Autodesk Fusion 360 part; units mm, degrees
(part 2 of 8)
  line L10 (6.9913, -88.2838) -> (6.7749, -88.3028)
  line L11 (6.7749, -88.3028) -> (7.0246, -88.3098)
  spline S251 degree 3 poles (7.0246, -88.3098) (7.1657, -88.3126) (7.2814, -88.3135) (7.2879, -88.3052) knots 0 0 0 0 1 1 1 1
  spline S252 degree 3 poles (7.2879, -88.3052) (7.2923, -88.2996) (7.2762, -88.2915) (7.2558, -88.289) knots 0 0 0 0 1 1 1 1
  spline S253 degree 3 poles (7.2558, -88.289) (7.1973, -88.2836) (7.3015, -88.1904) (7.3872, -88.1723) knots 0 0 0 0 1 1 1 1
  spline S254 degree 3 poles (7.3872, -88.1723) (7.4801, -88.1509) (7.4384, -88.1183) (7.3122, -88.1137) knots 0 0 0 0 1 1 1 1
  spline S255 degree 3 poles (7.3122, -88.1137) (7.1931, -88.1057) (7.1743, -88.0552) (7.2799, -88.0347) knots 0 0 0 0 1 1 1 1
  spline S256 degree 3 poles (7.2799, -88.0347) (7.3507, -88.0185) (7.348, -88.0163) (7.2641, -88.009) knots 0 0 0 0 1 1 1 1
  spline S257 degree 3 poles (7.2641, -88.009) (7.2029, -88.0014) (7.1744, -88.015) (7.178, -88.0447) knots 0 0 0 0 1 1 1 1
  spline S258 degree 3 poles (7.178, -88.0447) (7.1878, -88.1239) (7.1686, -88.1313) (6.9508, -88.1178) knots 0 0 0 0 1 1 1 1
  spline S259 degree 3 poles (6.9508, -88.1178) (6.6934, -88.1092) (6.6114, -88.1168) (6.6162, -88.1564) knots 0 0 0 0 1 1 1 1
  spline S260 degree 3 poles (6.6162, -88.1564) (6.618, -88.1713) (6.5929, -88.1919) (6.5589, -88.2012) knots 0 0 0 0 1 1 1 1
  spline S261 degree 3 poles (6.5589, -88.2012) (6.5121, -88.2094) (6.5084, -88.2199) (6.5306, -88.2373) knots 0 0 0 0 1 1 1 1
  spline S262 degree 3 poles (3.0505, -92.9095) (3.0667, -92.9804) (3.0716, -92.9798) (3.0703, -92.9071) knots 0 0 0 0 1 1 1 1
  spline S263 degree 3 poles (3.0703, -92.9071) (3.0703, -92.8668) (3.0655, -92.8272) (3.0599, -92.8229) knots 0 0 0 0 1 1 1 1
  spline S264 degree 3 poles (3.0599, -92.8229) (3.0377, -92.8055) (3.0342, -92.8386) (3.0505, -92.9095) knots 0 0 0 0 1 1 1 1
  spline S265 degree 3 poles (6.6279, -88.3133) (6.6335, -88.3177) (6.6731, -88.3128) (6.7143, -88.3002) knots 0 0 0 0 1 1 1 1
  spline S266 degree 3 poles (6.7143, -88.3002) (6.783, -88.2867) (6.7824, -88.2818) (6.7097, -88.2832) knots 0 0 0 0 1 1 1 1
  spline S267 degree 3 poles (6.7097, -88.2832) (6.637, -88.2846) (6.6057, -88.2959) (6.6279, -88.3133) knots 0 0 0 0 1 1 1 1
  spline S268 degree 3 poles (3.0531, -93.1354) (3.0693, -93.2062) (3.0742, -93.2056) (3.0729, -93.1329) knots 0 0 0 0 1 1 1 1
  spline S269 degree 3 poles (3.0729, -93.1329) (3.0729, -93.0927) (3.0681, -93.0531) (3.0625, -93.0487) knots 0 0 0 0 1 1 1 1
  spline S270 degree 3 poles (3.0625, -93.0487) (3.0403, -93.0314) (3.0368, -93.0645) (3.0531, -93.1354) knots 0 0 0 0 1 1 1 1
  line L12 (3.0526, -93.3365) -> (3.0753, -93.4392)
  line L13 (3.0753, -93.4392) -> (3.0724, -93.334)
  spline S271 degree 3 poles (3.0724, -93.334) (3.068, -93.2366) (3.0588, -93.2025) (3.0414, -93.2248) knots 0 0 0 0 1 1 1 1
  spline S272 degree 3 poles (3.0414, -93.2248) (3.0371, -93.2303) (3.0431, -93.2798) (3.0526, -93.3365) knots 0 0 0 0 1 1 1 1
  line L14 (3.0552, -93.5623) -> (3.0779, -93.6651)
  line L15 (3.0779, -93.6651) -> (3.075, -93.5599)
  spline S273 degree 3 poles (3.075, -93.5599) (3.0706, -93.4624) (3.0614, -93.4284) (3.044, -93.4506) knots 0 0 0 0 1 1 1 1
  spline S274 degree 3 poles (3.044, -93.4506) (3.0397, -93.4562) (3.0457, -93.5057) (3.0552, -93.5623) knots 0 0 0 0 1 1 1 1
  spline S275 degree 3 poles (7.3742, -88.0458) (7.3798, -88.0501) (7.4194, -88.0452) (7.4606, -88.0326) knots 0 0 0 0 1 1 1 1
  spline S276 degree 3 poles (7.4606, -88.0326) (7.5293, -88.0192) (7.5287, -88.0142) (7.456, -88.0156) knots 0 0 0 0 1 1 1 1
  spline S277 degree 3 poles (7.456, -88.0156) (7.3832, -88.017) (7.352, -88.0284) (7.3742, -88.0458) knots 0 0 0 0 1 1 1 1
  spline S278 degree 3 poles (8.0494, -87.4451) (8.5983, -87.4531) (9.0302, -87.4504) (9.0389, -87.4392) knots 0 0 0 0 1 1 1 1
  spline S279 degree 3 poles (9.0389, -87.4392) (9.0519, -87.4226) (8.2342, -87.4149) (8.0151, -87.4317) knots 0 0 0 0 1 1 1 1
  spline S280 degree 3 poles (8.0151, -87.4317) (7.8582, -87.4435) (7.8582, -87.4435) (8.0494, -87.4451) knots 0 0 0 0 1 1 1 1
  spline S281 degree 3 poles (3.0548, -93.7635) (3.071, -93.8343) (3.076, -93.8337) (3.0746, -93.761) knots 0 0 0 0 1 1 1 1
  spline S282 degree 3 poles (3.0746, -93.761) (3.0747, -93.7208) (3.0698, -93.6812) (3.0642, -93.6768) knots 0 0 0 0 1 1 1 1
  spline S283 degree 3 poles (3.0642, -93.6768) (3.042, -93.6595) (3.0385, -93.6926) (3.0548, -93.7635) knots 0 0 0 0 1 1 1 1
  spline S284 degree 3 poles (7.3295, -88.2347) (7.3657, -88.2629) (7.5307, -88.2351) (7.5264, -88.2005) knots 0 0 0 0 1 1 1 1
  spline S285 degree 3 poles (7.5264, -88.2005) (7.5246, -88.1856) (7.5586, -88.1764) (7.601, -88.1737) knots 0 0 0 0 1 1 1 1
  spline S286 degree 3 poles (7.601, -88.1737) (7.6737, -88.1723) (7.6743, -88.1773) (7.6056, -88.1907) knots 0 0 0 0 1 1 1 1
  spline S287 degree 3 poles (7.6056, -88.1907) (7.5645, -88.2033) (7.5387, -88.2191) (7.5499, -88.2278) knots 0 0 0 0 1 1 1 1
  spline S288 degree 3 poles (7.5499, -88.2278) (7.5888, -88.2582) (7.9208, -88.24) (7.9243, -88.2069) knots 0 0 0 0 1 1 1 1
  spline S289 degree 3 poles (7.9243, -88.2069) (7.9274, -88.1915) (7.9729, -88.1733) (8.0308, -88.1737) knots 0 0 0 0 1 1 1 1
  line L16 (8.0308, -88.1737) -> (8.1332, -88.1687)
  line L17 (8.1332, -88.1687) -> (8.0326, -88.1886)
  spline S290 degree 3 poles (8.0326, -88.1886) (7.9738, -88.2008) (7.941, -88.2199) (7.9576, -88.233) knots 0 0 0 0 1 1 1 1
  spline S291 degree 3 poles (7.9576, -88.233) (7.9938, -88.2612) (8.1588, -88.2334) (8.1545, -88.1988) knots 0 0 0 0 1 1 1 1
  spline S292 degree 3 poles (8.1545, -88.1988) (8.1527, -88.1839) (8.1867, -88.1747) (8.2291, -88.172) knots 0 0 0 0 1 1 1 1
  spline S293 degree 3 poles (8.2291, -88.172) (8.3018, -88.1706) (8.3025, -88.1756) (8.2337, -88.189) knots 0 0 0 0 1 1 1 1
  spline S294 degree 3 poles (8.2337, -88.189) (8.1415, -88.2154) (8.1844, -88.2579) (8.28, -88.2386) knots 0 0 0 0 1 1 1 1
  spline S295 degree 3 poles (8.28, -88.2386) (8.3169, -88.2316) (8.3376, -88.2165) (8.3265, -88.2078) knots 0 0 0 0 1 1 1 1
  spline S296 degree 3 poles (8.3265, -88.2078) (8.3154, -88.1991) (8.3362, -88.184) (8.373, -88.177) knots 0 0 0 0 1 1 1 1
  spline S297 degree 3 poles (8.373, -88.177) (8.5247, -88.1433) (8.354, -88.1039) (8.0885, -88.1114) knots 0 0 0 0 1 1 1 1
  spline S298 degree 3 poles (8.0885, -88.1114) (7.5476, -88.1275) (7.4678, -88.1323) (7.4708, -88.157) knots 0 0 0 0 1 1 1 1
  spline S299 degree 3 poles (7.4708, -88.157) (7.4726, -88.1719) (7.4348, -88.1916) (7.3853, -88.1977) knots 0 0 0 0 1 1 1 1
  spline S300 degree 3 poles (7.3853, -88.1977) (7.3386, -88.2059) (7.3129, -88.2217) (7.3295, -88.2347) knots 0 0 0 0 1 1 1 1
  spline S301 degree 3 poles (7.8269, -88.1711) (7.8996, -88.1697) (7.9002, -88.1747) (7.8315, -88.1881) knots 0 0 0 0 1 1 1 1
  spline S302 degree 3 poles (7.8315, -88.1881) (7.7903, -88.2007) (7.7507, -88.2056) (7.7452, -88.2013) knots 0 0 0 0 1 1 1 1
  spline S303 degree 3 poles (7.7452, -88.2013) (7.7229, -88.1839) (7.7542, -88.1725) (7.8269, -88.1711) knots 0 0 0 0 1 1 1 1
  spline S304 degree 3 poles (4.7594, -91.5988) (4.7733, -91.6097) (4.798, -91.6067) (4.8089, -91.5928) knots 0 0 0 0 1 1 1 1
  spline S305 degree 3 poles (4.8089, -91.5928) (4.8219, -91.5761) (4.8167, -91.5541) (4.8028, -91.5433) knots 0 0 0 0 1 1 1 1
  spline S306 degree 3 poles (4.8028, -91.5433) (4.7861, -91.5302) (4.7663, -91.5327) (4.7533, -91.5493) knots 0 0 0 0 1 1 1 1
  spline S307 degree 3 poles (4.7533, -91.5493) (4.7424, -91.5632) (4.7427, -91.5858) (4.7594, -91.5988) knots 0 0 0 0 1 1 1 1
  spline S308 degree 3 poles (7.5506, -88.0492) (7.5561, -88.0536) (7.5957, -88.0487) (7.6369, -88.0361) knots 0 0 0 0 1 1 1 1
  spline S309 degree 3 poles (7.6369, -88.0361) (7.7056, -88.0227) (7.705, -88.0177) (7.6323, -88.0191) knots 0 0 0 0 1 1 1 1
  spline S310 degree 3 poles (7.6323, -88.0191) (7.5596, -88.0205) (7.5283, -88.0319) (7.5506, -88.0492) knots 0 0 0 0 1 1 1 1
  spline S311 degree 3 poles (3.0513, -93.9398) (3.0675, -94.0107) (3.0725, -94.0101) (3.0711, -93.9374) knots 0 0 0 0 1 1 1 1
  spline S312 degree 3 poles (3.0711, -93.9374) (3.0712, -93.8972) (3.0663, -93.8575) (3.0608, -93.8532) knots 0 0 0 0 1 1 1 1
  spline S313 degree 3 poles (3.0608, -93.8532) (3.0385, -93.8358) (3.0351, -93.8689) (3.0513, -93.9398) knots 0 0 0 0 1 1 1 1
  spline S314 degree 3 poles (6.5586, -89.4679) (6.5725, -89.4787) (6.5973, -89.4757) (6.6103, -89.459) knots 0 0 0 0 1 1 1 1
  spline S315 degree 3 poles (6.6103, -89.459) (6.6211, -89.4451) (6.6116, -89.4287) (6.5912, -89.4262) knots 0 0 0 0 1 1 1 1
  spline S316 degree 3 poles (6.5912, -89.4262) (6.568, -89.4215) (6.546, -89.4267) (6.5395, -89.435) knots 0 0 0 0 1 1 1 1
  spline S317 degree 3 poles (6.5395, -89.435) (6.5351, -89.4406) (6.5419, -89.4548) (6.5586, -89.4679) knots 0 0 0 0 1 1 1 1
  line L18 (3.0509, -94.1409) -> (3.0735, -94.2437)
  line L19 (3.0735, -94.2437) -> (3.0707, -94.1385)
  spline S318 degree 3 poles (3.0707, -94.1385) (3.0661, -94.0812) (3.0601, -94.0317) (3.0545, -94.0274) knots 0 0 0 0 1 1 1 1
  spline S319 degree 3 poles (3.0545, -94.0274) (3.0323, -94.01) (3.0316, -94.0453) (3.0509, -94.1409) knots 0 0 0 0 1 1 1 1
  spline S320 degree 3 poles (7.7764, -88.0466) (7.782, -88.051) (7.8216, -88.0461) (7.8628, -88.0335) knots 0 0 0 0 1 1 1 1
  spline S321 degree 3 poles (7.8628, -88.0335) (7.9315, -88.02) (7.9309, -88.0151) (7.8582, -88.0165) knots 0 0 0 0 1 1 1 1
  spline S322 degree 3 poles (7.8582, -88.0165) (7.7855, -88.0179) (7.7542, -88.0293) (7.7764, -88.0466) knots 0 0 0 0 1 1 1 1
  spline S323 degree 3 poles (6.2415, -90.1602) (6.2554, -90.1711) (6.2801, -90.1681) (6.2932, -90.1514) knots 0 0 0 0 1 1 1 1
  spline S324 degree 3 poles (6.2932, -90.1514) (6.304, -90.1375) (6.2945, -90.1211) (6.2741, -90.1185) knots 0 0 0 0 1 1 1 1
  spline S325 degree 3 poles (6.2741, -90.1185) (6.2509, -90.1139) (6.2289, -90.1191) (6.2224, -90.1274) knots 0 0 0 0 1 1 1 1
  spline S326 degree 3 poles (6.2224, -90.1274) (6.218, -90.133) (6.2248, -90.1472) (6.2415, -90.1602) knots 0 0 0 0 1 1 1 1
  line L20 (3.0535, -94.3668) -> (3.0761, -94.4696)
  line L21 (3.0761, -94.4696) -> (3.0733, -94.3644)
  spline S327 degree 3 poles (3.0733, -94.3644) (3.0688, -94.2669) (3.0596, -94.2328) (3.0423, -94.2551) knots 0 0 0 0 1 1 1 1
  spline S328 degree 3 poles (3.0423, -94.2551) (3.0379, -94.2606) (3.044, -94.3102) (3.0535, -94.3668) knots 0 0 0 0 1 1 1 1
  spline S329 degree 3 poles (5.2813, -91.4694) (5.2869, -91.4738) (5.3265, -91.4689) (5.3677, -91.4563) knots 0 0 0 0 1 1 1 1
  spline S330 degree 3 poles (5.3677, -91.4563) (5.4364, -91.4428) (5.4358, -91.4379) (5.3631, -91.4393) knots 0 0 0 0 1 1 1 1
  spline S331 degree 3 poles (5.3631, -91.4393) (5.2904, -91.4407) (5.2591, -91.452) (5.2813, -91.4694) knots 0 0 0 0 1 1 1 1
  spline S332 degree 3 poles (3.053, -94.5679) (3.0693, -94.6388) (3.0742, -94.6382) (3.0728, -94.5655) knots 0 0 0 0 1 1 1 1
  spline S333 degree 3 poles (3.0728, -94.5655) (3.0729, -94.5253) (3.0681, -94.4856) (3.0625, -94.4813) knots 0 0 0 0 1 1 1 1
  spline S334 degree 3 poles (3.0625, -94.4813) (3.0403, -94.4639) (3.0368, -94.497) (3.053, -94.5679) knots 0 0 0 0 1 1 1 1
  spline S335 degree 3 poles (7.913, -88.4219) (7.9835, -88.4233) (8.0485, -88.4204) (8.0529, -88.4148) knots 0 0 0 0 1 1 1 1
  spline S336 degree 3 poles (8.0529, -88.4148) (8.0594, -88.4065) (8.0074, -88.3927) (7.9412, -88.3858) knots 0 0 0 0 1 1 1 1
  spline S337 degree 3 poles (7.9412, -88.3858) (7.8744, -88.3739) (7.8122, -88.379) (7.8014, -88.3929) knots 0 0 0 0 1 1 1 1
  spline S338 degree 3 poles (7.8014, -88.3929) (7.7905, -88.4068) (7.8397, -88.4184) (7.913, -88.4219) knots 0 0 0 0 1 1 1 1
  spline S339 degree 3 poles (8.1787, -88.0475) (8.1842, -88.0519) (8.2238, -88.047) (8.265, -88.0344) knots 0 0 0 0 1 1 1 1
  spline S340 degree 3 poles (8.265, -88.0344) (8.3337, -88.0209) (8.3331, -88.016) (8.2604, -88.0174) knots 0 0 0 0 1 1 1 1
  spline S341 degree 3 poles (8.2604, -88.0174) (8.1877, -88.0188) (8.1564, -88.0301) (8.1787, -88.0475) knots 0 0 0 0 1 1 1 1
  spline S342 degree 3 poles (3.0526, -94.769) (3.0642, -94.8229) (3.0744, -94.8443) (3.0785, -94.8161) knots 0 0 0 0 1 1 1 1
  spline S343 degree 3 poles (3.0785, -94.8161) (3.0819, -94.783) (3.117, -94.7611) (3.1671, -94.76) knots 0 0 0 0 1 1 1 1
  spline S344 degree 3 poles (3.1671, -94.76) (3.2475, -94.7602) (3.2447, -94.758) (3.1646, -94.7402) knots 0 0 0 0 1 1 1 1
  spline S345 degree 3 poles (3.1646, -94.7402) (3.1183, -94.7308) (3.0722, -94.7038) (3.0648, -94.6846) knots 0 0 0 0 1 1 1 1
  spline S346 degree 3 poles (3.0648, -94.6846) (3.0387, -94.6149) (3.0321, -94.6635) (3.0526, -94.769) knots 0 0 0 0 1 1 1 1
  spline S347 degree 3 poles (7.786, -88.6361) (7.7999, -88.6469) (7.833, -88.6504) (7.8522, -88.643) knots 0 0 0 0 1 1 1 1
  spline S348 degree 3 poles (7.8522, -88.643) (7.8735, -88.6329) (7.8794, -88.6196) (7.8628, -88.6065) knots 0 0 0 0 1 1 1 1
  spline S349 degree 3 poles (7.8628, -88.6065) (7.8489, -88.5957) (7.8179, -88.5894) (7.7966, -88.5996) knots 0 0 0 0 1 1 1 1
  spline S350 degree 3 poles (7.7966, -88.5996) (7.7774, -88.607) (7.7693, -88.623) (7.786, -88.6361) knots 0 0 0 0 1 1 1 1
  spline S351 degree 3 poles (3.0521, -94.9701) (3.0684, -95.041) (3.0733, -95.0404) (3.0719, -94.9677) knots 0 0 0 0 1 1 1 1
  spline S352 degree 3 poles (3.0719, -94.9677) (3.072, -94.9275) (3.0672, -94.8879) (3.0616, -94.8835) knots 0 0 0 0 1 1 1 1
  spline S353 degree 3 poles (3.0616, -94.8835) (3.0394, -94.8662) (3.0359, -94.8993) (3.0521, -94.9701) knots 0 0 0 0 1 1 1 1
  spline S354 degree 3 poles (8.4045, -88.0449) (8.4101, -88.0492) (8.4497, -88.0444) (8.4909, -88.0318) knots 0 0 0 0 1 1 1 1
  spline S355 degree 3 poles (8.4909, -88.0318) (8.5596, -88.0183) (8.559, -88.0134) (8.4863, -88.0148) knots 0 0 0 0 1 1 1 1
  spline S356 degree 3 poles (8.4863, -88.0148) (8.4136, -88.0162) (8.3823, -88.0275) (8.4045, -88.0449) knots 0 0 0 0 1 1 1 1
  spline S357 degree 3 poles (8.3515, -88.2273) (8.3877, -88.2556) (8.9505, -88.2342) (8.9546, -88.2061) knots 0 0 0 0 1 1 1 1
  spline S358 degree 3 poles (8.9546, -88.2061) (8.955, -88.1884) (8.9934, -88.1737) (9.0364, -88.1759) knots 0 0 0 0 1 1 1 1
  spline S359 degree 3 poles (9.0364, -88.1759) (9.1063, -88.1724) (9.1069, -88.1773) (9.0382, -88.1908) knots 0 0 0 0 1 1 1 1
  spline S360 degree 3 poles (9.0382, -88.1908) (8.9921, -88.204) (8.9741, -88.2213) (8.9908, -88.2343) knots 0 0 0 0 1 1 1 1
  spline S361 degree 3 poles (8.9908, -88.2343) (9.0213, -88.2582) (9.1071, -88.2401) (9.1397, -88.1984) knots 0 0 0 0 1 1 1 1
  spline S362 degree 3 poles (9.1397, -88.1984) (9.1483, -88.1873) (9.2474, -88.1751) (9.3603, -88.1738) knots 0 0 0 0 1 1 1 1
  line L22 (9.3603, -88.1738) -> (9.5614, -88.1743)
  line L23 (9.5614, -88.1743) -> (9.3473, -88.1905)
  spline S363 degree 3 poles (9.3473, -88.1905) (9.0808, -88.2107) (9.1055, -88.2479) (9.376, -88.2398) knots 0 0 0 0 1 1 1 1
  spline S364 degree 3 poles (9.376, -88.2398) (9.4988, -88.2373) (9.5838, -88.2545) (9.5952, -88.2857) knots 0 0 0 0 1 1 1 1
  spline S365 degree 3 poles (9.5952, -88.2857) (9.606, -88.3121) (9.6165, -88.3158) (9.6113, -88.2938) knots 0 0 0 0 1 1 1 1
  spline S366 degree 3 poles (9.6113, -88.2938) (9.611, -88.2712) (9.6482, -88.2466) (9.6977, -88.2405) knots 0 0 0 0 1 1 1 1
  spline S367 degree 3 poles (9.6977, -88.2405) (9.7445, -88.2322) (9.7702, -88.2165) (9.7591, -88.2078) knots 0 0 0 0 1 1 1 1
  spline S368 degree 3 poles (9.7591, -88.2078) (9.748, -88.1991) (9.7786, -88.1828) (9.8303, -88.1739) knots 0 0 0 0 1 1 1 1
  spline S369 degree 3 poles (9.8303, -88.1739) (9.9755, -88.1486) (9.888, -88.1116) (9.7085, -88.1236) knots 0 0 0 0 1 1 1 1
  spline S370 degree 3 poles (9.7085, -88.1236) (9.6209, -88.1268) (9.5405, -88.1266) (9.5294, -88.1179) knots 0 0 0 0 1 1 1 1
  spline S371 degree 3 poles (9.5294, -88.1179) (9.5183, -88.1092) (9.4802, -88.1063) (9.4455, -88.1106) knots 0 0 0 0 1 1 1 1
  spline S372 degree 3 poles (9.4455, -88.1106) (9.4109, -88.1149) (9.3057, -88.1177) (9.2098, -88.1144) knots 0 0 0 0 1 1 1 1
  spline S373 degree 3 poles (9.2098, -88.1144) (9.1166, -88.1133) (8.974, -88.1182) (8.8969, -88.1252) knots 0 0 0 0 1 1 1 1
  spline S374 degree 3 poles (8.8969, -88.1252) (8.8171, -88.13) (8.7416, -88.1292) (8.7277, -88.1183) knots 0 0 0 0 1 1 1 1
  spline S375 degree 3 poles (8.7277, -88.1183) (8.7138, -88.1075) (8.694, -88.1099) (8.681, -88.1266) knots 0 0 0 0 1 1 1 1
  spline S376 degree 3 poles (8.681, -88.1266) (8.6701, -88.1405) (8.688, -88.1634) (8.7217, -88.1718) knots 0 0 0 0 1 1 1 1
  spline S377 degree 3 poles (8.7217, -88.1718) (8.756, -88.1852) (8.7749, -88.1955) (8.7622, -88.1945) knots 0 0 0 0 1 1 1 1
  spline S378 degree 3 poles (8.7622, -88.1945) (8.5722, -88.2028) (8.5187, -88.1968) (8.5917, -88.1777) knots 0 0 0 0 1 1 1 1
  spline S379 degree 3 poles (8.5917, -88.1777) (8.6456, -88.1661) (8.6565, -88.1522) (8.6342, -88.1348) knots 0 0 0 0 1 1 1 1
  spline S380 degree 3 poles (8.6342, -88.1348) (8.5897, -88.1001) (8.4461, -88.1177) (8.451, -88.1573) knots 0 0 0 0 1 1 1 1
  spline S381 degree 3 poles (8.451, -88.1573) (8.4528, -88.1722) (8.4277, -88.1929) (8.3937, -88.2021) knots 0 0 0 0 1 1 1 1
  spline S382 degree 3 poles (8.3937, -88.2021) (8.3618, -88.2085) (8.3432, -88.2208) (8.3515, -88.2273) knots 0 0 0 0 1 1 1 1
  spline S383 degree 3 poles (9.7263, -88.1867) (9.7281, -88.2016) (9.6885, -88.2064) (9.64, -88.1998) knots 0 0 0 0 1 1 1 1
  spline S384 degree 3 poles (9.64, -88.1998) (9.5534, -88.1904) (9.5555, -88.1876) (9.6369, -88.1751) knots 0 0 0 0 1 1 1 1
  spline S385 degree 3 poles (9.6369, -88.1751) (9.6864, -88.169) (9.7273, -88.174) (9.7263, -88.1867) knots 0 0 0 0 1 1 1 1
  line L24 (3.0517, -95.1713) -> (3.0744, -95.274)
  line L25 (3.0744, -95.274) -> (3.0715, -95.1688)
  spline S386 degree 3 poles (3.0715, -95.1688) (3.0671, -95.0713) (3.0579, -95.0373) (3.0405, -95.0595) knots 0 0 0 0 1 1 1 1
  spline S387 degree 3 poles (3.0405, -95.0595) (3.0362, -95.0651) (3.0422, -95.1146) (3.0517, -95.1713) knots 0 0 0 0 1 1 1 1
  spline S388 degree 3 poles (8.6304, -88.0423) (8.636, -88.0466) (8.6756, -88.0418) (8.7168, -88.0292) knots 0 0 0 0 1 1 1 1
  spline S389 degree 3 poles (8.7168, -88.0292) (8.7855, -88.0157) (8.7849, -88.0108) (8.7122, -88.0122) knots 0 0 0 0 1 1 1 1
  spline S390 degree 3 poles (8.7122, -88.0122) (8.6394, -88.0135) (8.6082, -88.0249) (8.6304, -88.0423) knots 0 0 0 0 1 1 1 1
  spline S391 degree 3 poles (9.1636, -87.4516) (9.2159, -87.4477) (9.2626, -87.4394) (9.2691, -87.4311) knots 0 0 0 0 1 1 1 1
  spline S392 degree 3 poles (9.2691, -87.4311) (9.2756, -87.4227) (9.2376, -87.4199) (9.1853, -87.4238) knots 0 0 0 0 1 1 1 1
  spline S393 degree 3 poles (9.1853, -87.4238) (9.133, -87.4277) (9.0862, -87.4359) (9.0797, -87.4443) knots 0 0 0 0 1 1 1 1
  spline S394 degree 3 poles (9.0797, -87.4443) (9.0732, -87.4526) (9.1113, -87.4555) (9.1636, -87.4516) knots 0 0 0 0 1 1 1 1
  spline S395 degree 3 poles (3.0513, -95.3724) (3.0675, -95.4433) (3.0725, -95.4426) (3.0711, -95.3699) knots 0 0 0 0 1 1 1 1
  spline S396 degree 3 poles (3.0711, -95.3699) (3.0712, -95.3297) (3.0663, -95.2901) (3.0607, -95.2858) knots 0 0 0 0 1 1 1 1
  spline S397 degree 3 poles (3.0607, -95.2858) (3.0385, -95.2684) (3.035, -95.3015) (3.0513, -95.3724) knots 0 0 0 0 1 1 1 1
  line L26 (3.0508, -95.5735) -> (3.0735, -95.6763)
  line L27 (3.0735, -95.6763) -> (3.0706, -95.571)
  spline S398 degree 3 poles (3.0706, -95.571) (3.0662, -95.4736) (3.057, -95.4395) (3.0396, -95.4618) knots 0 0 0 0 1 1 1 1
  spline S399 degree 3 poles (3.0396, -95.4618) (3.0353, -95.4673) (3.0414, -95.5168) (3.0508, -95.5735) knots 0 0 0 0 1 1 1 1
  spline S400 degree 3 poles (9.563, -87.4503) (9.7162, -87.4491) (9.861, -87.4413) (9.883, -87.4361) knots 0 0 0 0 1 1 1 1
  spline S401 degree 3 poles (9.883, -87.4361) (9.9043, -87.426) (9.7957, -87.4217) (9.6398, -87.4207) knots 0 0 0 0 1 1 1 1
  spline S402 degree 3 poles (9.6398, -87.4207) (9.4866, -87.422) (9.3418, -87.4297) (9.3199, -87.4349) knots 0 0 0 0 1 1 1 1
  spline S403 degree 3 poles (9.3199, -87.4349) (9.2985, -87.4451) (9.4071, -87.4493) (9.563, -87.4503) knots 0 0 0 0 1 1 1 1
  spline S404 degree 3 poles (6.5564, -91.1897) (6.6087, -91.1858) (6.6554, -91.1776) (6.6619, -91.1692) knots 0 0 0 0 1 1 1 1
  spline S405 degree 3 poles (6.6619, -91.1692) (6.6685, -91.1609) (6.6304, -91.158) (6.5781, -91.1619) knots 0 0 0 0 1 1 1 1
  spline S406 degree 3 poles (6.5781, -91.1619) (6.5258, -91.1658) (6.4791, -91.1741) (6.4726, -91.1824) knots 0 0 0 0 1 1 1 1
  spline S407 degree 3 poles (6.4726, -91.1824) (6.466, -91.1908) (6.5041, -91.1936) (6.5564, -91.1897) knots 0 0 0 0 1 1 1 1
  line L28 (3.0511, -95.8826) -> (3.0643, -96.072)
  line L29 (3.0643, -96.072) -> (3.0687, -95.8829)
  spline S408 degree 3 poles (3.0687, -95.8829) (3.0718, -95.7242) (3.0639, -95.6598) (3.0444, -95.6849) knots 0 0 0 0 1 1 1 1
  spline S409 degree 3 poles (3.0444, -95.6849) (3.0401, -95.6904) (3.0433, -95.778) (3.0511, -95.8826) knots 0 0 0 0 1 1 1 1
  spline S410 degree 3 poles (7.6583, -89.9913) (7.5611, -90.1616) (7.4813, -90.3096) (7.4853, -90.3217) knots 0 0 0 0 1 1 1 1
  spline S411 degree 3 poles (7.4853, -90.3217) (7.4898, -90.3789) (7.5413, -90.3073) (7.7112, -89.9924) knots 0 0 0 0 1 1 1 1
  spline S412 degree 3 poles (7.7112, -89.9924) (7.8137, -89.8038) (7.9144, -89.6407) (7.9363, -89.6355) knots 0 0 0 0 1 1 1 1
  spline S413 degree 3 poles (7.9363, -89.6355) (7.9577, -89.6253) (7.9543, -89.6182) (7.9289, -89.6163) knots 0 0 0 0 1 1 1 1
  spline S414 degree 3 poles (7.9289, -89.6163) (7.9008, -89.6122) (7.8701, -89.6285) (7.8571, -89.6452) knots 0 0 0 0 1 1 1 1
  spline S415 degree 3 poles (7.8571, -89.6452) (7.8447, -89.6668) (7.7555, -89.821) (7.6583, -89.9913) knots 0 0 0 0 1 1 1 1
  spline S416 degree 3 poles (8.9103, -88.5206) (8.9808, -88.522) (9.0437, -88.5219) (9.048, -88.5163) knots 0 0 0 0 1 1 1 1
  spline S417 degree 3 poles (9.048, -88.5163) (9.0523, -88.5107) (9.0026, -88.4942) (8.9385, -88.4845) knots 0 0 0 0 1 1 1 1
  spline S418 degree 3 poles (8.9385, -88.4845) (8.8717, -88.4726) (8.8117, -88.4749) (8.7987, -88.4916) knots 0 0 0 0 1 1 1 1
  spline S419 degree 3 poles (8.7987, -88.4916) (8.7878, -88.5055) (8.8348, -88.5199) (8.9103, -88.5206) knots 0 0 0 0 1 1 1 1
  spline S420 degree 3 poles (8.2573, -89.2819) (8.2809, -89.269) (8.2976, -89.2418) (8.2958, -89.2269) knots 0 0 0 0 1 1 1 1
  spline S421 degree 3 poles (8.2958, -89.2269) (8.2962, -89.2093) (8.2748, -89.2194) (8.2537, -89.2522) knots 0 0 0 0 1 1 1 1
  spline S422 degree 3 poles (8.2537, -89.2522) (8.2298, -89.2828) (8.2316, -89.2976) (8.2573, -89.2819) knots 0 0 0 0 1 1 1 1
  line L30 (3.0525, -96.2016) -> (3.0752, -96.3044)
  line L31 (3.0752, -96.3044) -> (3.0724, -96.1992)
  spline S423 degree 3 poles (3.0724, -96.1992) (3.0679, -96.1017) (3.0587, -96.0676) (3.0413, -96.0899) knots 0 0 0 0 1 1 1 1
  spline S424 degree 3 poles (3.0413, -96.0899) (3.037, -96.0954) (3.0431, -96.1449) (3.0525, -96.2016) knots 0 0 0 0 1 1 1 1
  spline S425 degree 3 poles (7.0702, -91.0764) (7.1374, -91.0706) (7.1962, -91.0584) (7.2006, -91.0528) knots 0 0 0 0 1 1 1 1
  spline S426 degree 3 poles (7.2006, -91.0528) (7.2071, -91.0445) (7.1591, -91.0428) (7.092, -91.0486) knots 0 0 0 0 1 1 1 1
  spline S427 degree 3 poles (7.092, -91.0486) (7.0248, -91.0543) (6.966, -91.0665) (6.9617, -91.0721) knots 0 0 0 0 1 1 1 1
  spline S428 degree 3 poles (6.9617, -91.0721) (6.9551, -91.0804) (7.0031, -91.0821) (7.0702, -91.0764) knots 0 0 0 0 1 1 1 1
  spline S429 degree 3 poles (4.765, -93.9983) (4.7724, -94.0175) (4.7906, -94.0228) (4.8015, -94.0089) knots 0 0 0 0 1 1 1 1
  spline S430 degree 3 poles (4.8015, -94.0089) (4.8145, -93.9922) (4.8115, -93.9675) (4.7976, -93.9566) knots 0 0 0 0 1 1 1 1
  spline S431 degree 3 poles (4.7976, -93.9566) (4.7809, -93.9436) (4.7654, -93.9405) (4.7611, -93.946) knots 0 0 0 0 1 1 1 1
  spline S432 degree 3 poles (4.7611, -93.946) (4.7546, -93.9544) (4.7548, -93.9769) (4.765, -93.9983) knots 0 0 0 0 1 1 1 1
  spline S433 degree 3 poles (9.9779, -87.4521) (10.4408, -87.4556) (10.9145, -87.4452) (10.921, -87.4368) knots 0 0 0 0 1 1 1 1
  spline S434 degree 3 poles (10.921, -87.4368) (10.9275, -87.4285) (10.7082, -87.4228) (10.4393, -87.4231) knots 0 0 0 0 1 1 1 1
  spline S435 degree 3 poles (10.4393, -87.4231) (10.1677, -87.4213) (9.9424, -87.4288) (9.9359, -87.4372) knots 0 0 0 0 1 1 1 1
  spline S436 degree 3 poles (9.9359, -87.4372) (9.9294, -87.4455) (9.9504, -87.453) (9.9779, -87.4521) knots 0 0 0 0 1 1 1 1
  spline S437 degree 3 poles (3.0521, -96.4027) (3.0684, -96.4736) (3.0733, -96.473) (3.0719, -96.4003) knots 0 0 0 0 1 1 1 1
  spline S438 degree 3 poles (3.0719, -96.4003) (3.072, -96.36) (3.0671, -96.3204) (3.0616, -96.3161) knots 0 0 0 0 1 1 1 1
  spline S439 degree 3 poles (3.0616, -96.3161) (3.0393, -96.2987) (3.0359, -96.3318) (3.0521, -96.4027) knots 0 0 0 0 1 1 1 1
  spline S440 degree 3 poles (8.9747, -88.7992) (9.0137, -88.7894) (9.0579, -88.8016) (9.0758, -88.8245) knots 0 0 0 0 1 1 1 1
  spline S441 degree 3 poles (9.0758, -88.8245) (9.1032, -88.8639) (9.1054, -88.8611) (9.0894, -88.8128) knots 0 0 0 0 1 1 1 1
  spline S442 degree 3 poles (9.0894, -88.8128) (9.0734, -88.7645) (9.1063, -88.7454) (9.2595, -88.704) knots 0 0 0 0 1 1 1 1
  spline S443 degree 3 poles (9.2595, -88.704) (9.5474, -88.6334) (9.5546, -88.63) (9.5379, -88.617) knots 0 0 0 0 1 1 1 1
  spline S444 degree 3 poles (9.5379, -88.617) (9.5156, -88.5996) (8.945, -88.7627) (8.9233, -88.7905) knots 0 0 0 0 1 1 1 1
  spline S445 degree 3 poles (8.9233, -88.7905) (8.9125, -88.8044) (8.9357, -88.8091) (8.9747, -88.7992) knots 0 0 0 0 1 1 1 1
  spline S446 degree 3 poles (7.3691, -90.9517) (7.4127, -90.9589) (7.4529, -90.959) (7.4594, -90.9507) knots 0 0 0 0 1 1 1 1
  spline S447 degree 3 poles (7.4594, -90.9507) (7.4638, -90.9451) (7.4344, -90.9311) (7.3908, -90.9239) knots 0 0 0 0 1 1 1 1
  spline S448 degree 3 poles (7.3908, -90.9239) (7.3472, -90.9167) (7.307, -90.9166) (7.3005, -90.9249) knots 0 0 0 0 1 1 1 1
  spline S449 degree 3 poles (7.3005, -90.9249) (7.2961, -90.9305) (7.3255, -90.9445) (7.3691, -90.9517) knots 0 0 0 0 1 1 1 1
  spline S450 degree 3 poles (7.3012, -91.0329) (7.3151, -91.0438) (7.3482, -91.0473) (7.3674, -91.0399) knots 0 0 0 0 1 1 1 1
  spline S451 degree 3 poles (7.3674, -91.0399) (7.3887, -91.0297) (7.3946, -91.0164) (7.378, -91.0034) knots 0 0 0 0 1 1 1 1
  spline S452 degree 3 poles (7.378, -91.0034) (7.3641, -90.9925) (7.3331, -90.9863) (7.3118, -90.9964) knots 0 0 0 0 1 1 1 1
  spline S453 degree 3 poles (7.3118, -90.9964) (7.2926, -91.0038) (7.2845, -91.0199) (7.3012, -91.0329) knots 0 0 0 0 1 1 1 1
  spline S454 degree 3 poles (10.0458, -87.5544) (10.0767, -87.5606) (10.1114, -87.5564) (10.1222, -87.5425) knots 0 0 0 0 1 1 1 1
  spline S455 degree 3 poles (10.1222, -87.5425) (10.1353, -87.5258) (10.1164, -87.5155) (10.0762, -87.5154) knots 0 0 0 0 1 1 1 1
  spline S456 degree 3 poles (10.0762, -87.5154) (10.0387, -87.5175) (10.0041, -87.5218) (9.9997, -87.5273) knots 0 0 0 0 1 1 1 1
  spline S457 degree 3 poles (9.9997, -87.5273) (9.9954, -87.5329) (10.017, -87.5453) (10.0458, -87.5544) knots 0 0 0 0 1 1 1 1
  line L32 (3.0517, -96.6038) -> (3.0743, -96.7066)
  line L33 (3.0743, -96.7066) -> (3.0715, -96.6014)
  spline S458 degree 3 poles (3.0715, -96.6014) (3.067, -96.5441) (3.0609, -96.4946) (3.0553, -96.4903) knots 0 0 0 0 1 1 1 1
  spline S459 degree 3 poles (3.0553, -96.4903) (3.0331, -96.4729) (3.0324, -96.5082) (3.0517, -96.6038) knots 0 0 0 0 1 1 1 1
  spline S460 degree 3 poles (3.0512, -96.8049) (3.0675, -96.8758) (3.0724, -96.8752) (3.071, -96.8025) knots 0 0 0 0 1 1 1 1
  spline S461 degree 3 poles (3.071, -96.8025) (3.0711, -96.7623) (3.0663, -96.7227) (3.0607, -96.7183) knots 0 0 0 0 1 1 1 1
  spline S462 degree 3 poles (3.0607, -96.7183) (3.0385, -96.7009) (3.035, -96.734) (3.0512, -96.8049) knots 0 0 0 0 1 1 1 1
  spline S463 degree 3 poles (9.8371, -88.0449) (9.8426, -88.0493) (9.8823, -88.0444) (9.9234, -88.0318) knots 0 0 0 0 1 1 1 1
  spline S464 degree 3 poles (9.9234, -88.0318) (9.9922, -88.0184) (9.9915, -88.0134) (9.9188, -88.0148) knots 0 0 0 0 1 1 1 1
  spline S465 degree 3 poles (9.9188, -88.0148) (9.8461, -88.0162) (9.8148, -88.0276) (9.8371, -88.0449) knots 0 0 0 0 1 1 1 1
  spline S466 degree 3 poles (8.3907, -89.9994) (8.4185, -90.0211) (8.432, -90.0496) (8.4255, -90.058) knots 0 0 0 0 1 1 1 1
  spline S467 degree 3 poles (8.4255, -90.058) (8.419, -90.0663) (8.359, -90.1717) (8.291, -90.2931) knots 0 0 0 0 1 1 1 1
  spline S468 degree 3 poles (8.291, -90.2931) (8.1323, -90.5765) (8.0293, -90.9661) (8.0302, -91.2802) knots 0 0 0 0 1 1 1 1
  line L34 (8.0302, -91.2802) -> (8.0337, -91.5336)
  line L35 (8.0337, -91.5336) -> (7.9077, -91.5516)
  spline S469 degree 3 poles (7.9077, -91.5516) (7.8384, -91.5601) (7.7731, -91.5807) (7.7644, -91.5918) knots 0 0 0 0 1 1 1 1
  spline S470 degree 3 poles (7.7644, -91.5918) (7.7535, -91.6057) (7.8114, -91.6061) (7.89, -91.5914) knots 0 0 0 0 1 1 1 1
  line L36 (7.89, -91.5914) -> (8.033, -91.5689)
  line L37 (8.033, -91.5689) -> (8.1002, -91.8094)
  spline S471 degree 3 poles (8.1002, -91.8094) (8.1524, -91.989) (8.1554, -92.054) (8.1089, -92.0848) knots 0 0 0 0 1 1 1 1
  spline S472 degree 3 poles (8.1089, -92.0848) (8.0745, -92.1117) (8.0714, -92.1271) (8.0995, -92.1312) knots 0 0 0 0 1 1 1 1
  spline S473 degree 3 poles (8.0995, -92.1312) (8.1861, -92.1407) (8.2018, -92.0634) (8.1474, -91.8866) knots 0 0 0 0 1 1 1 1
  spline S474 degree 3 poles (8.1474, -91.8866) (8.0814, -91.6559) (8.0629, -91.4848) (8.0888, -91.3484) knots 0 0 0 0 1 1 1 1
  spline S475 degree 3 poles (8.0888, -91.3484) (8.0992, -91.2893) (8.0988, -91.2039) (8.0855, -91.1578) knots 0 0 0 0 1 1 1 1
  spline S476 degree 3 poles (8.0855, -91.1578) (8.0625, -91.0726) (8.1516, -90.6722) (8.1961, -90.6667) knots 0 0 0 0 1 1 1 1
  spline S477 degree 3 poles (8.1961, -90.6667) (8.211, -90.6649) (8.2194, -90.6311) (8.2167, -90.5888) knots 0 0 0 0 1 1 1 1
  spline S478 degree 3 poles (8.2167, -90.5888) (8.2168, -90.5485) (8.2672, -90.4267) (8.3371, -90.3201) knots 0 0 0 0 1 1 1 1
  line L38 (8.3371, -90.3201) -> (8.456, -90.1221)
  line L39 (8.456, -90.1221) -> (8.4579, -90.24)
  spline S479 degree 3 poles (8.4579, -90.24) (8.4577, -90.3204) (8.4192, -90.4156) (8.3341, -90.5417) knots 0 0 0 0 1 1 1 1
  spline S480 degree 3 poles (8.3341, -90.5417) (8.2658, -90.6405) (8.2136, -90.7475) (8.2179, -90.7821) knots 0 0 0 0 1 1 1 1
  spline S481 degree 3 poles (8.2179, -90.7821) (8.2255, -90.8239) (8.2342, -90.8128) (8.2675, -90.7358) knots 0 0 0 0 1 1 1 1
  spline S482 degree 3 poles (8.2675, -90.7358) (8.2933, -90.6799) (8.4233, -90.4905) (8.5629, -90.3175) knots 0 0 0 0 1 1 1 1
  spline S483 degree 3 poles (8.5629, -90.3175) (8.8003, -90.0195) (8.8319, -89.9905) (9.0887, -89.8509) knots 0 0 0 0 1 1 1 1
  spline S484 degree 3 poles (9.0887, -89.8509) (9.6001, -89.5744) (10.0678, -89.5145) (10.621, -89.6602) knots 0 0 0 0 1 1 1 1
  spline S485 degree 3 poles (10.621, -89.6602) (10.8752, -89.7245) (10.9633, -89.7665) (11.2321, -89.9496) knots 0 0 0 0 1 1 1 1
  spline S486 degree 3 poles (11.2321, -89.9496) (11.4931, -90.1312) (11.5225, -90.1452) (11.4194, -90.0422) knots 0 0 0 0 1 1 1 1
  spline S487 degree 3 poles (11.4194, -90.0422) (11.2499, -89.8695) (10.8651, -89.6629) (10.5982, -89.5977) knots 0 0 0 0 1 1 1 1
  line L40 (10.5982, -89.5977) -> (10.3756, -89.5446)
  line L41 (10.3756, -89.5446) -> (10.3755, -89.4415)
  spline S488 degree 3 poles (10.3755, -89.4415) (10.3759, -89.3837) (10.3819, -89.3302) (10.3884, -89.3218) knots 0 0 0 0 1 1 1 1
  spline S489 degree 3 poles (10.3884, -89.3218) (10.3971, -89.3107) (10.5054, -89.3326) (10.6325, -89.3647) knots 0 0 0 0 1 1 1 1
  line L42 (10.6325, -89.3647) -> (10.8635, -89.4243)
  line L43 (10.8635, -89.4243) -> (10.8663, -89.5296)
  line L44 (10.8663, -89.5296) -> (10.8664, -89.6326)
  line L45 (10.8664, -89.6326) -> (10.8858, -89.5448)
  spline S490 degree 3 poles (10.8858, -89.5448) (10.8974, -89.4956) (10.9194, -89.4502) (10.9371, -89.4505) knots 0 0 0 0 1 1 1 1
  spline S491 degree 3 poles (10.9371, -89.4505) (10.9569, -89.4481) (11.1302, -89.57) (11.3248, -89.7221) knots 0 0 0 0 1 1 1 1
  spline S492 degree 3 poles (11.3248, -89.7221) (11.5833, -89.9241) (11.6858, -90.0221) (11.6975, -90.0759) knots 0 0 0 0 1 1 1 1
  spline S493 degree 3 poles (11.6975, -90.0759) (11.7073, -90.1149) (11.718, -90.1413) (11.7246, -90.1329) knots 0 0 0 0 1 1 1 1
  spline S494 degree 3 poles (11.7246, -90.1329) (11.7311, -90.1246) (11.7894, -90.2104) (11.8535, -90.3232) knots 0 0 0 0 1 1 1 1
  spline S495 degree 3 poles (11.8535, -90.3232) (12.0064, -90.5859) (12.127, -91.0159) (12.0957, -91.1705) knots 0 0 0 0 1 1 1 1
  spline S496 degree 3 poles (12.0957, -91.1705) (12.0838, -91.2374) (12.0816, -91.2804) (12.0924, -91.2665) knots 0 0 0 0 1 1 1 1
  spline S497 degree 3 poles (12.0924, -91.2665) (12.1229, -91.2275) (12.1129, -91.5153) (12.0789, -91.6677) knots 0 0 0 0 1 1 1 1
  spline S498 degree 3 poles (12.0789, -91.6677) (12.0442, -91.8152) (12.0791, -91.8336) (12.1166, -91.6882) knots 0 0 0 0 1 1 1 1
  spline S499 degree 3 poles (12.1166, -91.6882) (12.136, -91.6004) (12.1496, -91.5887) (12.2273, -91.5867) knots 0 0 0 0 1 1 1 1
  spline S500 degree 3 poles (12.2273, -91.5867) (12.3099, -91.5841) (12.3099, -91.5841) (12.2326, -91.5684) knots 0 0 0 0 1 1 1 1
  spline S501 degree 3 poles (12.2326, -91.5684) (12.1602, -91.5522) (12.1488, -91.5209) (12.15, -91.2845) knots 0 0 0 0 1 1 1 1
  spline S502 degree 3 poles (12.15, -91.2845) (12.1485, -90.9655) (12.0435, -90.5612) (11.8894, -90.2886) knots 0 0 0 0 1 1 1 1
  spline S503 degree 3 poles (11.8894, -90.2886) (11.7375, -90.0132) (11.422, -89.6951) (11.1374, -89.5264) knots 0 0 0 0 1 1 1 1
  spline S504 degree 3 poles (11.1374, -89.5264) (10.9504, -89.4162) (10.9081, -89.3787) (10.912, -89.3279) knots 0 0 0 0 1 1 1 1
  spline S505 degree 3 poles (10.912, -89.3279) (10.9136, -89.28) (10.9108, -89.2778) (10.8915, -89.3254) knots 0 0 0 0 1 1 1 1
  spline S506 degree 3 poles (10.8915, -89.3254) (10.8638, -89.4067) (10.3879, -89.2767) (10.3946, -89.1879) knots 0 0 0 0 1 1 1 1
  spline S507 degree 3 poles (10.3946, -89.1879) (10.4018, -89.1443) (10.3885, -89.1383) (10.3452, -89.1537) knots 0 0 0 0 1 1 1 1
  spline S508 degree 3 poles (10.3452, -89.1537) (10.3139, -89.1651) (10.2845, -89.1913) (10.277, -89.2124) knots 0 0 0 0 1 1 1 1
  spline S509 degree 3 poles (10.277, -89.2124) (10.2695, -89.2334) (10.1931, -89.2453) (10.1071, -89.2408) knots 0 0 0 0 1 1 1 1
  spline S510 degree 3 poles (10.1071, -89.2408) (10.0211, -89.2362) (9.9273, -89.2302) (9.8948, -89.2316) knots 0 0 0 0 1 1 1 1
  spline S511 degree 3 poles (9.8948, -89.2316) (9.8568, -89.2288) (9.8327, -89.1965) (9.8165, -89.1257) knots 0 0 0 0 1 1 1 1
  line L46 (9.8165, -89.1257) -> (9.796, -89.0201)
  line L47 (9.796, -89.0201) -> (9.7976, -89.1154)
  spline S512 degree 3 poles (9.7976, -89.1154) (9.8015, -89.1677) (9.7955, -89.2212) (9.7868, -89.2323) knots 0 0 0 0 1 1 1 1
  spline S513 degree 3 poles (9.7868, -89.2323) (9.7673, -89.2574) (9.3097, -89.3789) (9.2931, -89.3658) knots 0 0 0 0 1 1 1 1
  spline S514 degree 3 poles (9.2931, -89.3658) (9.2847, -89.3593) (9.3027, -89.342) (9.3306, -89.3235) knots 0 0 0 0 1 1 1 1
  spline S515 degree 3 poles (9.3306, -89.3235) (9.3777, -89.2977) (9.3743, -89.2905) (9.3142, -89.2929) knots 0 0 0 0 1 1 1 1
  spline S516 degree 3 poles (9.3142, -89.2929) (9.2592, -89.2946) (9.2455, -89.3063) (9.2575, -89.3426) knots 0 0 0 0 1 1 1 1
  spline S517 degree 3 poles (9.2575, -89.3426) (9.2717, -89.376) (9.2193, -89.4201) (9.0666, -89.5068) knots 0 0 0 0 1 1 1 1
  spline S518 degree 3 poles (9.0666, -89.5068) (8.9073, -89.6017) (8.8491, -89.6189) (8.8118, -89.5808) knots 0 0 0 0 1 1 1 1
  spline S519 degree 3 poles (8.8118, -89.5808) (8.7716, -89.5405) (8.7695, -89.5432) (8.7817, -89.602) knots 0 0 0 0 1 1 1 1
  spline S520 degree 3 poles (8.7817, -89.602) (8.7887, -89.6389) (8.7685, -89.6992) (8.7325, -89.7337) knots 0 0 0 0 1 1 1 1
  spline S521 degree 3 poles (8.7325, -89.7337) (8.5027, -89.9706) (8.4569, -90.0064) (8.4037, -89.9827) knots 0 0 0 0 1 1 1 1
  spline S522 degree 3 poles (8.4037, -89.9827) (8.3505, -89.9591) (8.3484, -89.9619) (8.3907, -89.9994) knots 0 0 0 0 1 1 1 1
  spline S523 degree 3 poles (8.7689, -89.7846) (8.813, -89.7339) (8.813, -89.7339) (8.8251, -89.833) knots 0 0 0 0 1 1 1 1
  spline S524 degree 3 poles (8.8251, -89.833) (8.8389, -89.9243) (8.8199, -89.9542) (8.6729, -90.108) knots 0 0 0 0 1 1 1 1
  line L48 (8.6729, -90.108) -> (8.5079, -90.2791)
  line L49 (8.5079, -90.2791) -> (8.4924, -90.1729)
  spline S525 degree 3 poles (8.4924, -90.1729) (8.4787, -90.0816) (8.4905, -90.055) (8.6012, -89.9535) knots 0 0 0 0 1 1 1 1
  spline S526 degree 3 poles (8.6012, -89.9535) (8.6688, -89.8899) (8.745, -89.8151) (8.7689, -89.7846) knots 0 0 0 0 1 1 1 1
  spline S527 degree 3 poles (9.0838, -89.565) (9.2743, -89.4586) (9.3129, -89.4664) (9.2814, -89.5985) knots 0 0 0 0 1 1 1 1
  spline S528 degree 3 poles (9.2814, -89.5985) (9.263, -89.6736) (9.2248, -89.711) (9.0743, -89.7948) knots 0 0 0 0 1 1 1 1
  spline S529 degree 3 poles (9.0743, -89.7948) (8.9008, -89.8966) (8.8881, -89.8956) (8.8756, -89.8142) knots 0 0 0 0 1 1 1 1
  spline S530 degree 3 poles (8.8756, -89.8142) (8.8573, -89.7059) (8.8747, -89.6836) (9.0838, -89.565) knots 0 0 0 0 1 1 1 1
  spline S531 degree 3 poles (9.7675, -89.3202) (9.7845, -89.3156) (9.7977, -89.3617) (9.7923, -89.4202) knots 0 0 0 0 1 1 1 1
  spline S532 degree 3 poles (9.7923, -89.4202) (9.7831, -89.5294) (9.7788, -89.5349) (9.6239, -89.5841) knots 0 0 0 0 1 1 1 1
  spline S533 degree 3 poles (9.6239, -89.5841) (9.3698, -89.663) (9.3283, -89.6531) (9.3308, -89.5296) knots 0 0 0 0 1 1 1 1
  spline S534 degree 3 poles (9.3308, -89.5296) (9.3344, -89.4161) (9.3273, -89.4195) (9.7675, -89.3202) knots 0 0 0 0 1 1 1 1
  line L50 (10.1066, -89.2986) -> (10.3381, -89.3004)
  line L51 (10.3381, -89.3004) -> (10.3381, -89.4034)
  spline S535 degree 3 poles (10.3381, -89.4034) (10.3371, -89.4563) (10.3311, -89.5098) (10.3246, -89.5182) knots 0 0 0 0 1 1 1 1
  spline S536 degree 3 poles (10.3246, -89.5182) (10.3202, -89.5237) (10.2107, -89.5321) (10.0801, -89.5331) knots 0 0 0 0 1 1 1 1
  line L52 (10.0801, -89.5331) -> (9.8465, -89.5341)
  line L53 (9.8465, -89.5341) -> (9.8464, -89.4311)
  spline S537 degree 3 poles (9.8464, -89.4311) (9.8469, -89.3732) (9.8529, -89.3197) (9.8594, -89.3114) knots 0 0 0 0 1 1 1 1
  spline S538 degree 3 poles (9.8594, -89.3114) (9.8681, -89.3003) (9.9782, -89.2968) (10.1066, -89.2986) knots 0 0 0 0 1 1 1 1
  spline S539 degree 3 poles (9.7924, -88.2339) (9.8286, -88.2621) (9.9533, -88.2342) (10.0029, -88.1879) knots 0 0 0 0 1 1 1 1
  spline S540 degree 3 poles (10.0029, -88.1879) (10.0231, -88.1679) (10.0256, -88.1475) (10.0046, -88.14) knots 0 0 0 0 1 1 1 1
  spline S541 degree 3 poles (10.0046, -88.14) (9.9863, -88.1347) (9.9693, -88.1393) (9.9662, -88.1547) knots 0 0 0 0 1 1 1 1
  spline S542 degree 3 poles (9.9662, -88.1547) (9.9652, -88.1674) (9.9169, -88.1834) (9.8631, -88.1951) knots 0 0 0 0 1 1 1 1
  spline S543 degree 3 poles (9.8631, -88.1951) (9.8064, -88.2045) (9.7785, -88.223) (9.7924, -88.2339) knots 0 0 0 0 1 1 1 1
  line L54 (3.0508, -97.006) -> (3.0735, -97.1088)
  line L55 (3.0735, -97.1088) -> (3.0706, -97.0036)
  spline S544 degree 3 poles (3.0706, -97.0036) (3.0662, -96.9061) (3.057, -96.8721) (3.0396, -96.8943) knots 0 0 0 0 1 1 1 1
  spline S545 degree 3 poles (3.0396, -96.8943) (3.0352, -96.8999) (3.0413, -96.9494) (3.0508, -97.006) knots 0 0 0 0 1 1 1 1
  spline S546 degree 3 poles (8.091, -90.4861) (8.1049, -90.4969) (8.1297, -90.4939) (8.1427, -90.4772) knots 0 0 0 0 1 1 1 1
  spline S547 degree 3 poles (8.1427, -90.4772) (8.1536, -90.4633) (8.144, -90.4469) (8.1236, -90.4444) knots 0 0 0 0 1 1 1 1
  spline S548 degree 3 poles (8.1236, -90.4444) (8.1004, -90.4397) (8.0784, -90.4449) (8.0719, -90.4532) knots 0 0 0 0 1 1 1 1
  spline S549 degree 3 poles (8.0719, -90.4532) (8.0676, -90.4588) (8.0744, -90.473) (8.091, -90.4861) knots 0 0 0 0 1 1 1 1
  spline S550 degree 3 poles (7.2874, -91.6579) (7.2894, -91.7356) (7.307, -91.7761) (7.3327, -91.7604) knots 0 0 0 0 1 1 1 1
  spline S551 degree 3 poles (7.3327, -91.7604) (7.3534, -91.7453) (7.4061, -91.867) (7.4592, -92.0741) knots 0 0 0 0 1 1 1 1
  spline S552 degree 3 poles (7.4592, -92.0741) (7.515, -92.2834) (7.6126, -92.5253) (7.7183, -92.7108) knots 0 0 0 0 1 1 1 1
  spline S553 degree 3 poles (7.7183, -92.7108) (7.8391, -92.9171) (7.8794, -93.0203) (7.8528, -93.0487) knots 0 0 0 0 1 1 1 1
  spline S554 degree 3 poles (7.8528, -93.0487) (7.8304, -93.0715) (7.8236, -93.0975) (7.8375, -93.1084) knots 0 0 0 0 1 1 1 1
  spline S555 degree 3 poles (7.8375, -93.1084) (7.8514, -93.1192) (7.8755, -93.1112) (7.8929, -93.089) knots 0 0 0 0 1 1 1 1
  spline S556 degree 3 poles (7.8929, -93.089) (7.9255, -93.0473) (7.9255, -93.0473) (8.2839, -93.4079) knots 0 0 0 0 1 1 1 1
  spline S557 degree 3 poles (8.2839, -93.4079) (8.508, -93.6367) (8.966, -93.8871) (9.3646, -94.0015) knots 0 0 0 0 1 1 1 1
  spline S558 degree 3 poles (9.3646, -94.0015) (9.6151, -94.0763) (9.7026, -94.1134) (9.6997, -94.1514) knots 0 0 0 0 1 1 1 1
  spline S559 degree 3 poles (9.6997, -94.1514) (9.694, -94.1873) (9.7228, -94.1963) (9.7965, -94.1823) knots 0 0 0 0 1 1 1 1
  spline S560 degree 3 poles (9.7965, -94.1823) (9.8822, -94.1642) (9.8844, -94.1614) (9.8188, -94.1594) knots 0 0 0 0 1 1 1 1
  spline S561 degree 3 poles (9.8188, -94.1594) (9.7764, -94.1621) (9.7371, -94.1493) (9.7353, -94.1345) knots 0 0 0 0 1 1 1 1
  spline S562 degree 3 poles (9.7353, -94.1345) (9.7335, -94.1196) (9.8904, -94.1079) (10.0859, -94.104) knots 0 0 0 0 1 1 1 1
  spline S563 degree 3 poles (10.0859, -94.104) (10.5306, -94.1022) (11.0206, -93.9792) (11.366, -93.7834) knots 0 0 0 0 1 1 1 1
  spline S564 degree 3 poles (11.366, -93.7834) (11.5116, -93.7002) (11.6622, -93.6164) (11.7, -93.5967) knots 0 0 0 0 1 1 1 1
  spline S565 degree 3 poles (11.7, -93.5967) (11.7378, -93.577) (11.8844, -93.4408) (12.0271, -93.2926) knots 0 0 0 0 1 1 1 1
  spline S566 degree 3 poles (12.0271, -93.2926) (12.2302, -93.0842) (12.3208, -92.9625) (12.4515, -92.7379) knots 0 0 0 0 1 1 1 1
  spline S567 degree 3 poles (12.4515, -92.7379) (12.5854, -92.4977) (12.618, -92.456) (12.6514, -92.4821) knots 0 0 0 0 1 1 1 1
  spline S568 degree 3 poles (12.6514, -92.4821) (12.6708, -92.4973) (12.6984, -92.4964) (12.7092, -92.4825) knots 0 0 0 0 1 1 1 1
  spline S569 degree 3 poles (12.7092, -92.4825) (12.7223, -92.4659) (12.7115, -92.4395) (12.6821, -92.4255) knots 0 0 0 0 1 1 1 1
  spline S570 degree 3 poles (12.6821, -92.4255) (12.6206, -92.3954) (12.7798, -91.7677) (12.8429, -91.7901) knots 0 0 0 0 1 1 1 1
  spline S571 degree 3 poles (12.8429, -91.7901) (12.8639, -91.7975) (12.8908, -91.7917) (12.9038, -91.775) knots 0 0 0 0 1 1 1 1
  spline S572 degree 3 poles (12.9038, -91.775) (12.9169, -91.7584) (12.9045, -91.7398) (12.8758, -91.7307) knots 0 0 0 0 1 1 1 1
  spline S573 degree 3 poles (12.8758, -91.7307) (12.8498, -91.7239) (12.8236, -91.6944) (12.8211, -91.6746) knots 0 0 0 0 1 1 1 1
  spline S574 degree 3 poles (12.8211, -91.6746) (12.8181, -91.6498) (12.7903, -91.6281) (12.7522, -91.6253) knots 0 0 0 0 1 1 1 1
  spline S575 degree 3 poles (12.7522, -91.6253) (12.6944, -91.6248) (12.6944, -91.6248) (12.742, -91.6441) knots 0 0 0 0 1 1 1 1
  spline S576 degree 3 poles (12.742, -91.6441) (12.784, -91.6591) (12.7767, -91.7429) (12.7106, -91.9822) knots 0 0 0 0 1 1 1 1
  spline S577 degree 3 poles (12.7106, -91.9822) (12.6648, -92.1613) (12.6112, -92.2985) (12.5902, -92.2911) knots 0 0 0 0 1 1 1 1
  spline S578 degree 3 poles (12.5902, -92.2911) (12.5404, -92.2746) (12.5041, -92.3268) (12.5545, -92.3482) knots 0 0 0 0 1 1 1 1
  spline S579 degree 3 poles (12.5545, -92.3482) (12.6027, -92.3725) (12.2918, -92.9309) (12.2392, -92.9122) knots 0 0 0 0 1 1 1 1
  spline S580 degree 3 poles (12.2392, -92.9122) (12.221, -92.9069) (12.1941, -92.9127) (12.1832, -92.9266) knots 0 0 0 0 1 1 1 1
  spline S581 degree 3 poles (12.1832, -92.9266) (12.1702, -92.9433) (12.1819, -92.9569) (12.2073, -92.9589) knots 0 0 0 0 1 1 1 1
  spline S582 degree 3 poles (12.2073, -92.9589) (12.2404, -92.9623) (12.222, -92.9973) (12.1436, -93.0747) knots 0 0 0 0 1 1 1 1
  spline S583 degree 3 poles (12.1436, -93.0747) (12.0803, -93.1328) (11.9709, -93.2442) (11.8989, -93.3134) knots 0 0 0 0 1 1 1 1
  spline S584 degree 3 poles (11.8989, -93.3134) (11.8118, -93.402) (11.7532, -93.4368) (11.7282, -93.4173) knots 0 0 0 0 1 1 1 1
  spline S585 degree 3 poles (11.7282, -93.4173) (11.706, -93.3999) (11.6784, -93.4008) (11.6654, -93.4175) knots 0 0 0 0 1 1 1 1
  spline S586 degree 3 poles (11.6654, -93.4175) (11.6545, -93.4314) (11.6613, -93.4456) (11.6845, -93.4503) knots 0 0 0 0 1 1 1 1
  spline S587 degree 3 poles (11.6845, -93.4503) (11.7458, -93.4579) (11.725, -93.473) (11.4202, -93.6511) knots 0 0 0 0 1 1 1 1
  spline S588 degree 3 poles (11.4202, -93.6511) (11.1618, -93.7985) (10.506, -94.0248) (10.4482, -93.9841) knots 0 0 0 0 1 1 1 1
  spline S589 degree 3 poles (10.4482, -93.9841) (10.4343, -93.9732) (10.4473, -93.9566) (10.4737, -93.9458) knots 0 0 0 0 1 1 1 1
  spline S590 degree 3 poles (10.4737, -93.9458) (10.4978, -93.9378) (10.4768, -93.9303) (10.4195, -93.9348) knots 0 0 0 0 1 1 1 1
  spline S591 degree 3 poles (10.4195, -93.9348) (10.3645, -93.9366) (10.3162, -93.9526) (10.3158, -93.9702) knots 0 0 0 0 1 1 1 1
  spline S592 degree 3 poles (10.3158, -93.9702) (10.3117, -93.9984) (9.7956, -94.0115) (9.7595, -93.9832) knots 0 0 0 0 1 1 1 1
  spline S593 degree 3 poles (9.7595, -93.9832) (9.7511, -93.9767) (9.7867, -93.9598) (9.8434, -93.9503) knots 0 0 0 0 1 1 1 1
  line L56 (9.8434, -93.9503) -> (9.944, -93.9304)
  line L57 (9.944, -93.9304) -> (9.8283, -93.9295)
  spline S594 degree 3 poles (9.8283, -93.9295) (9.7599, -93.9254) (9.7193, -93.9429) (9.7267, -93.9621) knots 0 0 0 0 1 1 1 1
  spline S595 degree 3 poles (9.7267, -93.9621) (9.7421, -94.0055) (9.572, -93.9711) (9.2402, -93.8685) knots 0 0 0 0 1 1 1 1
  spline S596 degree 3 poles (9.2402, -93.8685) (9.0887, -93.8218) (9.0665, -93.8044) (9.0675, -93.7515) knots 0 0 0 0 1 1 1 1
  spline S597 degree 3 poles (9.0675, -93.7515) (9.0692, -93.7036) (9.0664, -93.7014) (9.0493, -93.7462) knots 0 0 0 0 1 1 1 1
  spline S598 degree 3 poles (9.0493, -93.7462) (9.0328, -93.796) (8.9885, -93.7838) (8.7966, -93.6742) knots 0 0 0 0 1 1 1 1
  spline S599 degree 3 poles (8.7966, -93.6742) (8.3214, -93.4058) (8.0015, -93.0932) (7.7463, -92.6521) knots 0 0 0 0 1 1 1 1
  spline S600 degree 3 poles (7.7463, -92.6521) (7.6097, -92.42) (7.5836, -92.3504) (7.6257, -92.3251) knots 0 0 0 0 1 1 1 1
  spline S601 degree 3 poles (7.6257, -92.3251) (7.6672, -92.2949) (7.6644, -92.2927) (7.6183, -92.3059) knots 0 0 0 0 1 1 1 1
  spline S602 degree 3 poles (7.6183, -92.3059) (7.5672, -92.3197) (7.5407, -92.2677) (7.4726, -91.9996) knots 0 0 0 0 1 1 1 1
  spline S603 degree 3 poles (7.4726, -91.9996) (7.4116, -91.7683) (7.4044, -91.6687) (7.4388, -91.6418) knots 0 0 0 0 1 1 1 1
  spline S604 degree 3 poles (7.4388, -91.6418) (7.4831, -91.6138) (7.4803, -91.6116) (7.4342, -91.6248) knots 0 0 0 0 1 1 1 1
  spline S605 degree 3 poles (7.4342, -91.6248) (7.4001, -91.634) (7.3663, -91.6658) (7.3579, -91.6995) knots 0 0 0 0 1 1 1 1
  spline S606 degree 3 poles (7.3579, -91.6995) (7.3445, -91.7338) (7.3294, -91.7131) (7.3169, -91.6317) knots 0 0 0 0 1 1 1 1
  spline S607 degree 3 poles (7.3169, -91.6317) (7.2903, -91.4766) (7.2767, -91.4883) (7.2874, -91.6579) knots 0 0 0 0 1 1 1 1
  spline S608 degree 3 poles (10.3901, -93.9611) (10.4105, -93.9636) (10.4201, -93.98) (10.4092, -93.9939) knots 0 0 0 0 1 1 1 1
  spline S609 degree 3 poles (10.4092, -93.9939) (10.3962, -94.0106) (10.3714, -94.0136) (10.3575, -94.0028) knots 0 0 0 0 1 1 1 1
  spline S610 degree 3 poles (10.3575, -94.0028) (10.3408, -93.9898) (10.334, -93.9755) (10.3384, -93.9699) knots 0 0 0 0 1 1 1 1
  spline S611 degree 3 poles (10.3384, -93.9699) (10.3449, -93.9616) (10.3669, -93.9564) (10.3901, -93.9611) knots 0 0 0 0 1 1 1 1
  spline S612 degree 3 poles (9.6555, -88.5925) (9.7585, -88.5924) (9.7613, -88.5946) (9.7077, -88.6288) knots 0 0 0 0 1 1 1 1
  spline S613 degree 3 poles (9.7077, -88.6288) (9.6727, -88.6507) (9.6646, -88.6668) (9.6928, -88.6709) knots 0 0 0 0 1 1 1 1
  spline S614 degree 3 poles (9.6928, -88.6709) (9.7181, -88.6728) (9.7432, -88.6521) (9.7501, -88.6261) knots 0 0 0 0 1 1 1 1
  spline S615 degree 3 poles (9.7501, -88.6261) (9.7591, -88.5974) (9.8322, -88.5783) (9.9127, -88.5785) knots 0 0 0 0 1 1 1 1
  spline S616 degree 3 poles (9.9127, -88.5785) (10.046, -88.5797) (10.1566, -88.5184) (10.101, -88.475) knots 0 0 0 0 1 1 1 1
  spline S617 degree 3 poles (10.101, -88.475) (10.0871, -88.4641) (10.0657, -88.4743) (10.0583, -88.4953) knots 0 0 0 0 1 1 1 1
  spline S618 degree 3 poles (10.0583, -88.4953) (10.0458, -88.5169) (9.9266, -88.5492) (9.7929, -88.5656) knots 0 0 0 0 1 1 1 1
  spline S619 degree 3 poles (9.7929, -88.5656) (9.6565, -88.5798) (9.5955, -88.5948) (9.6555, -88.5925) knots 0 0 0 0 1 1 1 1
  spline S620 degree 3 poles (9.8953, -88.3142) (9.9008, -88.3186) (9.9405, -88.3137) (9.9816, -88.3011) knots 0 0 0 0 1 1 1 1
  spline S621 degree 3 poles (9.9816, -88.3011) (10.0504, -88.2877) (10.0497, -88.2827) (9.977, -88.2841) knots 0 0 0 0 1 1 1 1
  spline S622 degree 3 poles (9.977, -88.2841) (9.9043, -88.2855) (9.873, -88.2969) (9.8953, -88.3142) knots 0 0 0 0 1 1 1 1
  line L58 (3.0534, -97.2319) -> (3.0761, -97.3347)
  line L59 (3.0761, -97.3347) -> (3.0732, -97.2295)